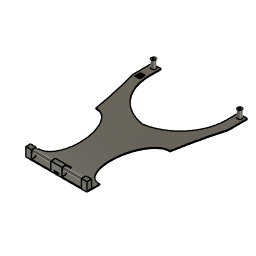
case-handle (Autodesk Fusion 360 design; units mm, degrees)
Autodesk Fusion 360 part; units mm, degrees
sketch "Esboço1" plane through (0, 0, 0) normal (0, 0, 1) x (1, 0, 0)
  line L0 (-52, 78) -> (52, 78)
  line L1 (52, 78) -> (52, -78)
  line L2 (52, -78) -> (-52, -78)
  line L3 (-52, -78) -> (-52, 78)
  dimension "d1" = 104
  dimension "d2" = 156
  dimension "d3" = 52
  dimension "d4" = 78
  constraint horizontal L0
  constraint vertical L1
  constraint horizontal L2
  constraint vertical L3
  measures "d1" distance of L0.start L0.end
  measures "d2" distance of L0.start L2.end
  measures "d3" distance of origin L1
  measures "d4" distance of origin L0
extrude "Extrusão1" add sketch "Esboço1" along normal blind 0.8
sketch "Esboço2" plane through (0, 0, 0.8) normal (0, 0, 1) x (-1, 0, 0)
  line L0 (52, 78) -> (-52, 78)
  line L1 (-52, 78) -> (-52, -78)
  line L2 (-52, -78) -> (52, -78)
  line L3 (52, -78) -> (52, 78)
  line L4 (-52, -78) -> (-42, -78)
  line L5 (-42, -78) -> (-42, -65)
  line L6 (-42, -65) -> (-52, -65)
  line L7 (-52, -65) -> (-52, -78)
  line L8 (0, -1.75) -> (0, -22.5)
  line L9 (42, -65) -> (52, -65)
  line L10 (42, -78) -> (42, -65)
  line L11 (52, -65) -> (52, -78)
  line L12 (52, -78) -> (42, -78)
  line L13 (42, -65) -> (-42, -65)
  line L14 (-42, -65) -> (-42, -78)
  line L15 (-42, -78) -> (42, -78)
  line L16 (42, -78) -> (42, -65)
  point P0 (52, -78)
  dimension "d7" = 10
  dimension "d8" = 13
  constraint horizontal L4
  constraint vertical L5
  constraint horizontal L6
  constraint vertical L7
  constraint coincident L1.end L2.start
  constraint symmetric L1.end L8 P0
  constraint symmetric L4.end L8 L10.start
  constraint symmetric L5.end L8 L9.start
  constraint symmetric L6.end L8 L9.end
  constraint horizontal L13
  constraint vertical L14
  constraint horizontal L15
  constraint vertical L16
  measures "d7" distance of L1.end L4.end
  measures "d8" distance of L1.end L6.end
extrude "Extrusão2" cut sketch "Esboço2" against normal blind 2 contours L2 L5 L10 L13 L14 L15 L16
sketch "Esboço3" plane through (0, 0, 0.8) normal (0, 0, 1) x (-1, 0, 0)
  line L0 (42, -65) -> (42, -78)
  line L1 (42, -78) -> (52, -78)
  line L2 (52, -78) -> (52, 78)
  line L3 (52, 78) -> (-52, 78)
  line L4 (-52, 78) -> (-52, -78)
  line L5 (-52, -78) -> (-42, -78)
  line L6 (-42, -78) -> (-42, -65)
  line L7 (-42, -65) -> (42, -65)
  line L8 (-33.25, 78) -> (33.25, 78)
  line L9 (33.25, 78) -> (33.25, 75)
  line L10 (33.25, 75) -> (-33.25, 75)
  line L11 (-33.25, 75) -> (-33.25, 78)
  arc A0 (33.25, 78) -> (52, -57.0483) centre (528.9728, 78) ccw
  line L12 (52, -57.0483) -> (52, 78)
  line L13 (0, -1.75) -> (0, -22.5)
  arc A1 (-52, -57.0483) -> (-33.25, 78) centre (-528.9728, 78) ccw
  line L14 (-33.25, 78) -> (-33.25, 75)
  line L15 (-52, -57.0483) -> (-52, 78)
  arc A2 (42, -65) -> (-0.2595, -15.5) centre (-8.1203, -65) ccw
  arc A3 (0.2595, -15.5) -> (-42, -65) centre (8.1203, -65) ccw
  point P0 (-52, 78)
  point P1 (-42, -65)
  point P2 (-0.2595, -15.5)
  dimension "d11" = 66.5
  dimension "d12" = 3
  dimension "d13" = 18.75
  dimension "d14" = 62.5
  constraint horizontal L8
  constraint vertical L9
  constraint horizontal L10
  constraint vertical L11
  constraint coincident L3 L8.start
  constraint coincident L2 A0.end
  constraint tangent L9 A0
  constraint coincident L2.end L3.start
  constraint symmetric L0.start L13 L6.end
  constraint symmetric L2.end L13 P0
  constraint symmetric L8.end L13 L8.start
  constraint symmetric L9.end L13 L10.end
  constraint symmetric A0.end L13 A1.start
  constraint symmetric A0 L13 A1
  constraint tangent L0 A2
  constraint coincident L0.start L7.end
  constraint coincident P2 A2.end
  constraint symmetric L13 L0.start P1
  constraint symmetric L13 P2 A3.start
  constraint symmetric L13 A2 A3
  measures "d11" distance of L8.start L8.end
  measures "d12" distance of L8.start L10.end
  measures "d13" distance of L4 L11
  measures "d14" distance of L1 P2
extrude "Extrusão3" cut sketch "Esboço3" against normal blind 2 contours L7 A2 A3 | L2 L3 A0 L12 | L3 L4 A1 L15
sketch "Esboço4" plane through (0, 0, 0.8) normal (0, 0, 1) x (-1, 0, 0)
  arc A0 (0, -15.5419) -> (-42, -65) centre (8.1203, -65) ccw
  arc A1 (42, -65) -> (0, -15.5419) centre (-8.1203, -65) ccw
  line L0 (42, -65) -> (42, -78)
  line L1 (42, -78) -> (52, -78)
  line L2 (52, -78) -> (52, -57.0483)
  arc A2 (33.25, 78) -> (52, -57.0483) centre (528.9728, 78) ccw
  line L3 (33.25, 78) -> (-33.25, 78)
  arc A3 (-52, -57.0483) -> (-33.25, 78) centre (-528.9728, 78) ccw
  line L4 (-52, -57.0483) -> (-52, -78)
  line L5 (-52, -78) -> (-42, -78)
  line L6 (-42, -78) -> (-42, -65)
  line L7 (-33.25, 78) -> (33.25, 78)
  line L8 (33.25, 78) -> (33.25, 73)
  line L9 (33.25, 73) -> (-33.25, 73)
  line L10 (-33.25, 73) -> (-33.25, 78)
  line L11 (-33.25, 78) -> (-27.25, 78)
  line L12 (-27.25, 78) -> (-27.25, 69)
  line L13 (-27.25, 69) -> (-33.25, 69)
  line L14 (-33.25, 69) -> (-33.25, 78)
  line L15 (33.25, 78) -> (27.25, 78)
  line L16 (27.25, 78) -> (27.25, 69)
  line L17 (27.25, 69) -> (33.25, 69)
  line L18 (33.25, 69) -> (33.25, 78)
  line L19 (-6, 78) -> (6, 78)
  line L20 (6, 78) -> (6, 69)
  line L21 (6, 69) -> (-6, 69)
  line L22 (-6, 69) -> (-6, 78)
  dimension "d17" = 66.5
  dimension "d18" = 5
  dimension "d19" = 6
  dimension "d20" = 6
  dimension "d21" = 12
  dimension "d22" = 6
  constraint horizontal L7
  constraint vertical L8
  constraint horizontal L9
  constraint vertical L10
  constraint coincident L3.end A3.end
  constraint horizontal L11
  constraint vertical L12
  constraint horizontal L13
  constraint vertical L14
  constraint horizontal L15
  constraint vertical L16
  constraint horizontal L17
  constraint vertical L18
  constraint coincident A2.start L3.start
  constraint horizontal L19
  constraint vertical L20
  constraint horizontal L21
  constraint vertical L22
  constraint coincident L7 L19.start
  measures "d17" distance of L3.end A2.start
  measures "d18" distance of L3.end L9.end
  measures "d19" distance of L3.end L11.end
  measures "d20" distance of A2.start L15.end
  measures "d21" distance of L19.start L19.end
  measures "d22" distance of origin L20
extrude "Extrusão4" add sketch "Esboço4" along normal blind 9 contours L3 L7 L9 L10 L11 L12 L14 | L3 L7 L8 L9 L15 L16 L18 | L3 L7 L9 L19 L20 L22
sketch "Esboço5" plane through (-27.25, 0, 0) normal (1, 0, 0) x (0, 1, 0)
  line L0 (-78, 0.8) -> (-73, 0.8)
  line L1 (-73, 0.8) -> (-73, 9.8)
  line L2 (-73, 9.8) -> (-78, 9.8)
  circle A0 centre (-75.5, 7.8) radius 1.95
  line L3 (-78, 9.8) -> (-78, 0.8)
  point P0 (-75.5, 7.8)
  dimension "d25" = 2
  dimension "d27" = 3.9
  dimension "d43" = 2.5
  constraint coincident P0 A0.centre
  measures "d25" distance of L2 P0
  measures "d27" diameter of A0
  measures "d43" distance of P0 L3
extrude "Extrusão5" add sketch "Esboço5" along normal blind 60.5 contours A0
sketch "Esboço6" plane through (0, 0, 0.8) normal (0, 0, 1) x (-1, 0, 0)
  line L0 (-27.25, 78) -> (-27.25, 73)
  line L1 (-27.25, 73) -> (-33.25, 73)
  line L2 (-33.25, 73) -> (-33.25, 78)
  arc A0 (-52, -57.0483) -> (-33.25, 78) centre (-528.9728, 78) ccw
  line L3 (-52, -57.0483) -> (-52, -78)
  line L4 (-52, -78) -> (-42, -78)
  line L5 (-42, -78) -> (-42, -65)
  arc A1 (0, -15.5419) -> (-42, -65) centre (8.1203, -65) ccw
  arc A2 (42, -65) -> (0, -15.5419) centre (-8.1203, -65) ccw
  line L6 (42, -65) -> (42, -78)
  line L7 (42, -78) -> (52, -78)
  line L8 (52, -78) -> (52, -57.0483)
  arc A3 (33.25, 78) -> (52, -57.0483) centre (528.9728, 78) ccw
  line L9 (33.25, 78) -> (33.25, 73)
  line L10 (33.25, 73) -> (27.25, 73)
  line L11 (27.25, 73) -> (27.25, 78)
  line L12 (27.25, 78) -> (6, 78)
  line L13 (6, 78) -> (6, 73)
  line L14 (6, 73) -> (-6, 73)
  line L15 (-6, 73) -> (-6, 78)
  line L16 (-6, 78) -> (-27.25, 78)
  circle A4 centre (-47, -74.75) radius 2.375
  line L17 (0, -1.75) -> (0, -22.5)
  circle A5 centre (47, -74.75) radius 2.375
  point P0 (-47, -74.75)
  point P1 (47, -74.75)
  point P2 (52, -57.0483)
  point P3 (52, -78)
  point P4 (42, -78)
  point P5 (42, -65)
  dimension "d30" = 5
  dimension "d31" = 3.25
  dimension "d32" = 4.75
  constraint coincident P0 A4.centre
  constraint symmetric A0.start L17 P2
  constraint symmetric L3.end L17 P3
  constraint symmetric L4.end L17 P4
  constraint symmetric L5.end L17 P5
  constraint symmetric P0 L17 P1
  constraint symmetric A4 L17 A5
  measures "d30" distance of L3 P0
  measures "d31" distance of L4 P0
  measures "d32" diameter of A4
extrude "Extrusão6" add sketch "Esboço6" along normal blind 8.5 contours A4 | A5
sketch "Esboço7" plane through (0, 0, 9.3) normal (0, 0, 1) x (-1, 0, 0)
  circle A0 centre (-47, -74.75) radius 2.375
  circle A1 centre (-47, -74.75) radius 0.75
  line L0 (0, -1.75) -> (0, -22.5)
  circle A2 centre (47, -74.75) radius 0.75
  point P0 (47, -74.75)
  dimension "d36" = 1.5
  dimension "d37" = 1.625
  constraint concentric A0 A1
  constraint symmetric A0.centre L0 P0
  constraint symmetric A1 L0 A2
  measures "d36" diameter of A1
  measures "d37" distance of A0 A1
extrude "Extrusão7" cut sketch "Esboço7" against normal blind 6 contours A1 | A2
sketch "Esboço8" plane through (0, 0, 0.8) normal (0, 0, 1) x (-1, 0, 0)
  circle A0 centre (47, -74.75) radius 2.375
  circle A1 centre (-47, -74.75) radius 2.375
  line L0 (-27.25, 78) -> (-27.25, 73)
  line L1 (-27.25, 73) -> (-33.25, 73)
  line L2 (-33.25, 73) -> (-33.25, 78)
  arc A2 (-52, -57.0483) -> (-33.25, 78) centre (-528.9728, 78) ccw
  line L3 (-52, -57.0483) -> (-52, -78)
  line L4 (-52, -78) -> (-42, -78)
  line L5 (-42, -78) -> (-42, -65)
  arc A3 (0, -15.5419) -> (-42, -65) centre (8.1203, -65) ccw
  arc A4 (42, -65) -> (0, -15.5419) centre (-8.1203, -65) ccw
  line L6 (42, -65) -> (42, -78)
  line L7 (42, -78) -> (52, -78)
  line L8 (52, -78) -> (52, -57.0483)
  arc A5 (33.25, 78) -> (52, -57.0483) centre (528.9728, 78) ccw
  line L9 (33.25, 78) -> (33.25, 73)
  line L10 (33.25, 73) -> (27.25, 73)
  line L11 (27.25, 73) -> (27.25, 78)
  line L12 (27.25, 78) -> (6, 78)
  line L13 (6, 78) -> (6, 73)
  line L14 (6, 73) -> (-6, 73)
  line L15 (-6, 73) -> (-6, 78)
  line L16 (-6, 78) -> (-27.25, 78)
  ellipse E0 centre (35.6344, 29.437) end of major axis (30.9782, 64.1259) minor radius 18.4551
  line L17 (40.2907, -5.2519) -> (30.9782, 64.1259) construction
  line L18 (53.9255, 31.8922) -> (17.3434, 26.9818) construction
  line L19 (0, -1.75) -> (0, -22.5)
  ellipse E1 centre (-35.6344, 29.437) end of major axis (-30.9782, 64.1259) minor radius 18.4551
  dimension "d42" = 70
  constraint coincident E0 L17.start
  constraint coincident E0 L17.end
  constraint coincident E0 L18.start
  constraint coincident E0 L18.end
  constraint coincident A5 E0.centre
  constraint symmetric E0 L19 E1
  constraint coincident A5 L17.start
  measures "d42" distance of E0
extrude "Extrusão8" cut sketch "Esboço8" against normal blind 10 contours A2 E1 | A5 E0 picked at (-29.7614, 27.7315) picked at (29.5401, 29.38)
sketch "Esboço9" plane through (0, 0, 0.8) normal (0, 0, 1) x (-1, 0, 0)
  ellipse E0 centre (35.6344, 29.437) end of major axis (30.9782, 64.1259) minor radius 18.4551 (33.4436, 64.1453) -> (40.2907, -5.2519) ccw
  arc A0 (33.25, 78) -> (33.4436, 64.1453) centre (528.9728, 78) ccw
  line L0 (33.25, 78) -> (33.25, 73)
  line L1 (33.25, 73) -> (27.25, 73)
  line L2 (27.25, 73) -> (27.25, 78)
  line L3 (27.25, 78) -> (6, 78)
  line L4 (6, 78) -> (6, 73)
  line L5 (6, 73) -> (-6, 73)
  line L6 (-6, 73) -> (-6, 78)
  line L7 (-6, 78) -> (-27.25, 78)
  line L8 (-27.25, 78) -> (-27.25, 73)
  line L9 (-27.25, 73) -> (-33.25, 73)
  line L10 (-33.25, 73) -> (-33.25, 78)
  arc A1 (-33.4436, 64.1453) -> (-33.25, 78) centre (-528.9728, 78) ccw
  ellipse E1 centre (-35.6344, 29.437) end of major axis (-30.9782, 64.1259) minor radius 18.4551 (-40.2907, -5.2519) -> (-33.4436, 64.1453) ccw
  arc A2 (-52, -57.0483) -> (-40.2907, -5.2519) centre (-528.9728, 78) ccw
  line L11 (-52, -57.0483) -> (-52, -78)
  line L12 (-52, -78) -> (-42, -78)
  line L13 (-42, -78) -> (-42, -65)
  arc A3 (0, -15.5419) -> (-42, -65) centre (8.1203, -65) ccw
  arc A4 (42, -65) -> (0, -15.5419) centre (-8.1203, -65) ccw
  line L14 (42, -65) -> (42, -78)
  line L15 (42, -78) -> (52, -78)
  line L16 (52, -78) -> (52, -57.0483)
  arc A5 (40.2907, -5.2519) -> (52, -57.0483) centre (528.9728, 78) ccw
  circle A6 centre (-47, -74.75) radius 2.375
  circle A7 centre (47, -74.75) radius 2.375
  line L17 (49.5, -63) -> (44.5, -63)
  line L18 (44.5, -63) -> (44.5, -61)
  line L19 (44.5, -61) -> (49.5, -61)
  line L20 (49.5, -61) -> (49.5, -63)
  line L21 (44.5, -59) -> (49.5, -59)
  line L22 (49.5, -59) -> (49.5, -57)
  line L23 (49.5, -57) -> (44.5, -57)
  line L24 (44.5, -57) -> (44.5, -59)
  line L25 (2.5, 70) -> (-2.5, 70)
  line L26 (-2.5, 70) -> (-2.5, 68)
  line L27 (-2.5, 68) -> (2.5, 68)
  line L28 (2.5, 68) -> (2.5, 70)
  line L29 (2.5, 66) -> (-2.5, 66)
  line L30 (-2.5, 66) -> (-2.5, 64)
  line L31 (-2.5, 64) -> (2.5, 64)
  line L32 (2.5, 64) -> (2.5, 66)
  dimension "d44" = 5
  dimension "d45" = 2
  dimension "d46" = 2.5
  dimension "d47" = 2.5
  dimension "d48" = 15
  dimension "d49" = 2.5
  dimension "d50" = 2
  dimension "d51" = 2
  dimension "d52" = 5
  dimension "d53" = 5
  dimension "d54" = 2
  dimension "d55" = 12
  dimension "d56" = 3.5
  dimension "d57" = 3
  dimension "d58" = 5
  dimension "d59" = 2
  dimension "d60" = 2
  constraint horizontal L17
  constraint vertical L18
  constraint horizontal L19
  constraint vertical L20
  constraint horizontal L21
  constraint vertical L22
  constraint horizontal L23
  constraint vertical L24
  constraint horizontal L25
  constraint vertical L26
  constraint horizontal L27
  constraint vertical L28
  constraint horizontal L29
  constraint vertical L30
  constraint horizontal L31
  constraint vertical L32
  measures "d44" distance of L18 L20
  measures "d45" distance of L17 L19
  measures "d46" distance of L14 L18
  measures "d47" distance of L16 L20
  measures "d48" distance of L15 L17
  measures "d49" distance of L16 L22
  measures "d50" distance of L19 L21
  measures "d51" distance of L21 L23
  measures "d52" distance of L22 L24
  measures "d53" distance of L25.start L25.end
  measures "d54" distance of L25.start L27.end
  measures "d55" distance of L4 L6
  measures "d56" distance of L6 L26
  measures "d57" distance of L5 L25
  measures "d58" distance of L29.start L29.end
  measures "d59" distance of L29.start L31.end
  measures "d60" distance of L27 L29
extrude "Extrusão9" cut sketch "Esboço9" against normal blind 0.4 contours L17 L18 L19 L20 | L21 L22 L23 L24 | L25 L26 L27 L28 | L29 L30 L31 L32
sketch "Esboço10" plane through (0, 61, 0) normal (0, 1, 0) x (-1, 0, 0)
  line L0 (49.5, 0.8) -> (44.5, 0.8)
  line L1 (44.5, 0.8) -> (44.5, 0.4)
  line L2 (44.5, 0.4) -> (49.5, 0.4)
  line L3 (49.5, 0.4) -> (49.5, 0.8)
  line L4 (44.5, 0.4) -> (49.5, 0.4)
  line L5 (49.5, 0.4) -> (49.5, 0.6)
  line L6 (49.5, 0.6) -> (44.5, 0.6)
  line L7 (44.5, 0.6) -> (44.5, 0.4)
  dimension "d63" = 5
  constraint horizontal L4
  constraint vertical L5
  constraint horizontal L6
  constraint vertical L7
  constraint coincident L1.end L2.start
  measures "d63" distance of L1.end L2.end
extrude "Extrusão10" cut sketch "Esboço10" against normal blind 2 contours L1 L2 L3 L4 L5 L6 L7
sketch "Esboço11" plane through (0, -73, 0) normal (0, 1, 0) x (-1, 0, 0)
  line L0 (-6, 0.8) -> (6, 0.8)
  line L1 (6, 0.8) -> (6, 9.8)
  line L2 (6, 9.8) -> (-6, 9.8)
  line L3 (-6, 9.8) -> (-6, 0.8)
  line L4 (-2.5, 1.5) -> (2.5, 1.5)
  line L5 (2.5, 1.5) -> (2.5, 2.5)
  line L6 (2.5, 2.5) -> (-2.5, 2.5)
  line L7 (-2.5, 2.5) -> (-2.5, 1.5)
  dimension "d66" = 1
  dimension "d67" = 5
  dimension "d68" = 3.5
  constraint horizontal L4
  constraint vertical L5
  constraint horizontal L6
  constraint vertical L7
  measures "d66" distance of L4.start L6.end
  measures "d67" distance of L5 L7
  measures "d68" distance of L1 L5
extrude "Extrusão11" cut sketch "Esboço11" against normal blind 20 contours L4 L5 L6 L7
sketch "Esboço12" plane through (0, -66, 0) normal (0, 1, 0) x (-1, 0, 0)
  line L0 (2.5, 0.8) -> (-2.5, 0.8)
  line L1 (-2.5, 0.8) -> (-2.5, 0.4)
  line L2 (-2.5, 0.4) -> (2.5, 0.4)
  line L3 (2.5, 0.4) -> (2.5, 0.8)
  line L4 (-2.5, 0.4) -> (2.5, 0.4)
  line L5 (2.5, 0.4) -> (2.5, 0.6)
  line L6 (2.5, 0.6) -> (-2.5, 0.6)
  line L7 (-2.5, 0.6) -> (-2.5, 0.4)
  dimension "d71" = 5
  constraint horizontal L4
  constraint vertical L5
  constraint horizontal L6
  constraint vertical L7
  constraint coincident L1.end L2.start
  measures "d71" distance of L1.end L2.end
extrude "Extrusão12" cut sketch "Esboço12" against normal blind 2 contours L1 L2 L3 L4 L5 L6 L7
equation "d2 = 148 mm + 8 mm"
equation "d3 = ( 104 / 2 ) * 1 mm"
equation "d4 = ( ( 148 + 8 ) / 2 ) * 1 mm"
equation "d13 = ( ( 104 - 66.5 ) / 2 ) * 1 mm"
equation "d22 = ( 12 / 2 ) * 1 mm"
equation "d28 = 66.5 mm - 6 mm"
